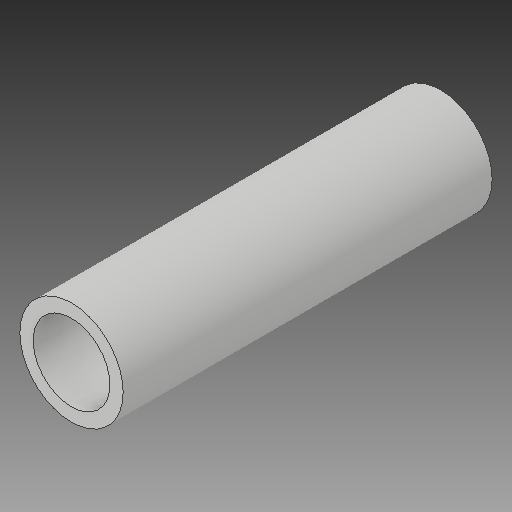
# Autodesk Inventor part: 25mmspacer
Saved by Autodesk Inventor 2018 (Build 220112000, 112)
## iProperties
Created: 2016-07-22
Part Number: 25mmspacer
Material: Generic
Document SubType Name: Modeling
Designer: User
Density: 1 g/cm^3
Appearance: Default
Mass: 0.431184 g
Surface Area: 9.9268 cm^2
Volume: 0.431184 cm^3
Author: User
Autodesk Inventor part; units mm, degrees
ref_plane "YZ Plane" through (0, 0, 0) normal (1, 0, 0) x (0, 1, 0)
ref_plane "XZ Plane" through (0, 0, 0) normal (0, 1, 0) x (-1, 0, 0)
ref_plane "XY Plane" through (0, 0, 0) normal (0, 0, 1) x (1, 0, 0)
sketch "Sketch1" plane through (0, 0, 0) normal (0, 0, 1) x (1, 0, 0)
  circle A0 centre (1.7813, 12.6893) radius 2.5 projected
  circle A1 centre (1.7813, 12.6893) radius 2.6
  circle A2 centre (1.7813, 12.6893) radius 3.5
  point P0 (0, 0)
  dimension "d0" = 5.2
  dimension "d1" = 7
  constraints: 2 centre point, 2 coincident
  measures "d0" diameter of A1
  measures "d1" diameter of A2
extrude "Extrusion1" add sketch "Sketch1" along normal blind 25 contours A2
body "Solid1"
